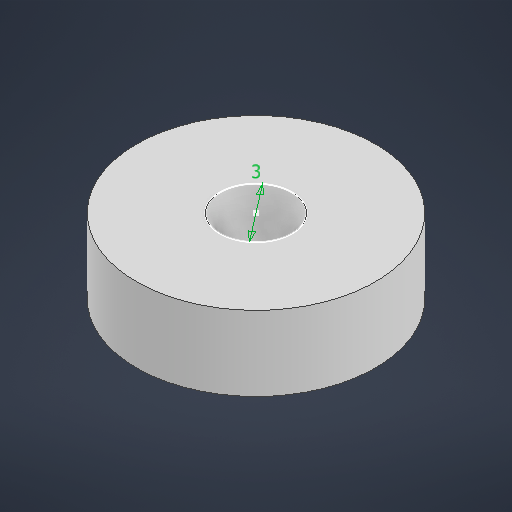
# Autodesk Inventor part: Acoustic Horn 45deg V1
Saved by Autodesk Inventor 2026 (Build 300175050, 175E)
## iProperties
Created: 2025-06-27
Part Number: Acoustic Horn 45deg V1
Material: Generic
Document SubType Name: Modeling
Designer: STW
Density: 1 g/cm^3
Appearance: Default
Author: STW
Autodesk Inventor part; units mm, degrees
ref_plane "YZ Plane" through (0, 0, 0) normal (1, 0, 0) x (0, 1, 0)
ref_plane "XZ Plane" through (0, 0, 0) normal (0, 1, 0) x (-1, 0, 0)
ref_plane "XY Plane" through (0, 0, 0) normal (0, 0, 1) x (1, 0, 0)
sketch "Sketch1" plane through (0, 0, 0) normal (0, 1, 0) x (-1, 0, 0)
  circle A0 centre (0, 0) radius 0.36
  circle A1 centre (0, 0) radius 5
  dimension "d0" = 0.72
  dimension "d2" = 10
  constraints: 2 centre point, 1 coincident, 1 concentric
  measures "d0" diameter of A0
  measures "d2" diameter of A1
extrude "Extrusion1" add sketch "Sketch1" along normal blind 3.125
sketch "Sketch2" plane through (0, 3.125, 0) normal (0, 1, 0) x (1, 0, 0)
  circle A0 centre (0, 0) radius 1.5
  dimension "d10" = 3
  constraints: 1 centre point, 1 coincident
  measures "d10" diameter of A0
sketch "Sketch3" plane through (0, 0, 0) normal (0, -1, 0) x (1, 0, 0)
  line L0 (-1.775, 1.775) -> (1.775, 1.775)
  line L1 (1.775, 1.775) -> (1.775, -1.775)
  line L2 (1.775, -1.775) -> (-1.775, -1.775)
  line L3 (-1.775, -1.775) -> (-1.775, 1.775)
  line L4 (-1.775, 1.775) -> (1.775, -1.775) construction
  line L5 (1.775, 1.775) -> (-1.775, -1.775) construction
  arc A0 (1.775, 1.475) -> (1.475, 1.775) centre (1.775, 1.775) ccw
  arc A1 (1.475, -1.775) -> (1.775, -1.475) centre (1.775, -1.775) ccw
  arc A2 (-1.775, -1.475) -> (-1.475, -1.775) centre (-1.775, -1.775) ccw
  arc A3 (-1.475, 1.775) -> (-1.775, 1.475) centre (-1.775, 1.775) ccw
  point P0 (0, 0)
  dimension "d11" = 0.3
  dimension "d13" = 3.55
  constraints: 12 end point, 8 point on circle, 8 point on line, 4 centre point, 4 coincident, 3 equal radius, 2 midpoint, 2 parallel, 2 perpendicular, 1 horizontal
  measures "d11" radius of A0
  measures "d13" distance of L1.end L2.end
extrude "Extrusion2" cut sketch "Sketch3" against normal blind 1.275
sketch "Sketch5" plane through (0, 0, 0) normal (0, 0, 1) x (1, 0, 0)
  line L0 (-0.36, 1.275) -> (0.36, 1.275) projected
  line L1 (5, 3.125) -> (-5, 3.125) projected
  arc A0 (-0.36, 1.275) -> (-1.5, 3.125) centre (-11.1041, -4.0695) ccw
  line L2 (0, 1.275) -> (0, 3.125)
  line L3 (0.36, 1.275) -> (0, 1.275)
  line L4 (0.36, 3.125) -> (0.36, 1.275) projected
  line L5 (0.36, 3.125) -> (-1.5, 3.125)
  point P0 (0, 0)
  dimension "d17" = 1.5
  dimension "d23" = 12
  constraints: 6 end point, 3 point on line, 2 collinear, 2 midpoint, 2 point on circle, 1 centre point, 1 vertical
  measures "d17" distance of L2.end L5.end
  measures "d23" radius of A0
revolve "Revolution1" cut sketch "Sketch5" angle 360 about axis through (0, 1.275, 0) along (0, 1, 0) contours A0 L1 L2 L0
fillet "Fillet1" radius 0.05 1 edges at (0.36, 1.275, 0)
equation "\"d17\" = 0.5 * d10"
body "Solid1"
